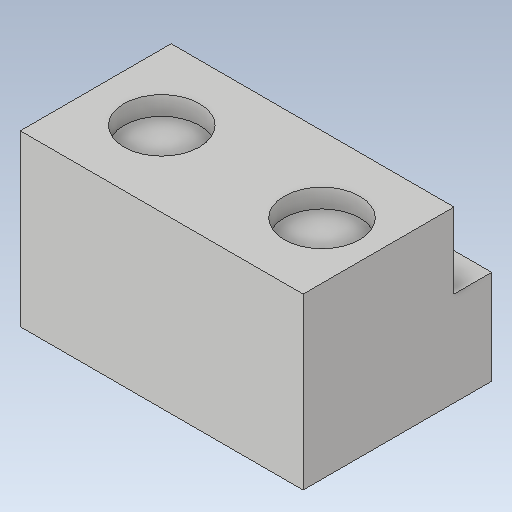
# Autodesk Inventor part: Sharp
Saved by Autodesk Inventor 2020 (Build 240168000, 168)
## iProperties
Created: 2019-01-30
Part Number: Sharp
Material: Ogólny
Document SubType Name: Modeling
Designer: atmat
Density: 1 g/cm^3
Appearance: Domyślna
Author: atmat
Autodesk Inventor part; units mm, degrees
ref_plane "YZ Plane" through (0, 0, 0) normal (1, 0, 0) x (0, 1, 0)
ref_plane "XZ Plane" through (0, 0, 0) normal (0, 1, 0) x (-1, 0, 0)
ref_plane "XY Plane" through (0, 0, 0) normal (0, 0, 1) x (1, 0, 0)
sketch "Szkic1" plane through (0, 0, 0) normal (0, 1, 0) x (-1, 0, 0)
  line L0 (7.5, 5) -> (-7.5, 5)
  line L1 (-7.5, 5) -> (-7.5, -5)
  line L2 (-7.5, -5) -> (7.5, -5)
  line L3 (7.5, -5) -> (7.5, 5)
  point P0 (0, 0)
  dimension "d0" = 10
  dimension "d1" = 15
  dimension "d2" = 5
  dimension "d3" = 7.5
  constraints: 8 end point, 2 parallel, 1 horizontal, 1 perpendicular
  measures "d0" distance of L2.end L0.start
  measures "d1" distance of L1.end L2.end
  measures "d2" distance from line of point (0, 0) L2
  measures "d3" distance from line of point (0, 0) L3
extrude "Wyciągnięcie proste1" add sketch "Szkic1" along normal blind 5
sketch "Szkic2" plane through (0, 5, 0) normal (0, 1, 0) x (1, 0, 0)
  line L0 (-7.5, -5) -> (7.5, -5) projected
  line L1 (7.5, -5) -> (7.5, 5) projected
  line L2 (-7.5, -5) -> (7.5, -5)
  line L3 (7.5, -5) -> (7.5, 3)
  line L4 (7.5, 3) -> (-7.5, 3)
  line L5 (-7.5, 3) -> (-7.5, -5)
  point P0 (0, 0)
  dimension "d6" = 8
  constraints: 8 end point, 2 parallel, 1 horizontal, 1 perpendicular, 1 point on line
  measures "d6" distance between parallel lines of L0 L4
extrude "Wyciągnięcie proste2" add sketch "Szkic2" along normal blind 4
sketch "Szkic3" plane through (0, 9, 0) normal (0, 1, 0) x (1, 0, 0)
  circle A0 centre (-4, -1) radius 2
  line L0 (-7.5, 3) -> (-7.5, -5) projected
  line L1 (7.5, 3) -> (-7.5, 3) projected
  circle A1 centre (4.5, -1) radius 2
  line L2 (7.5, -5) -> (7.5, 3) projected
  point P0 (0, 0)
  dimension "d9" = 4
  dimension "d10" = 3.5
  dimension "d11" = 4
  dimension "d12" = 3
  dimension "d13" = 4
  dimension "d14" = 4
  constraints: 2 centre point
  measures "d9" diameter of A0
  measures "d10" distance from line of L0 A0.centre
  measures "d11" distance from line of L1 A0.centre
  measures "d12" distance from line of L2 A1.centre
  measures "d13" distance from line of L1 A1.centre
  measures "d14" diameter of A1
extrude "Wyciągnięcie proste3" cut sketch "Szkic3" against normal blind 1
